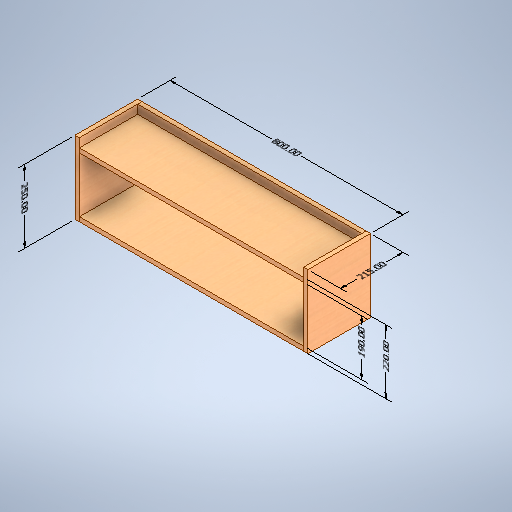
# Autodesk Inventor part: MM_00001.1.0
Saved by Autodesk Inventor 2025.3 (Build 293356000, 356)
## iProperties
Created: 2025-08-13
Part Number: MM_00001.1.0
Material: Wood (Cherry)
Document SubType Name: Modeling
Designer: FerreRo
Density: 0.63 g/cm^3
Appearance: Cherry - Natural Low Gloss
Author: FerreRo
Autodesk Inventor part; units mm, degrees
ref_plane "YZ Plane" through (0, 0, 0) normal (1, 0, 0) x (0, 1, 0)
ref_plane "XZ Plane" through (0, 0, 0) normal (0, 1, 0) x (-1, 0, 0)
ref_plane "XY Plane" through (0, 0, 0) normal (0, 0, 1) x (1, 0, 0)
sketch "Sketch1" plane through (0, 0, 0) normal (0, 0, 1) x (1, 0, 0)
  line L0 (-400, 125) -> (400, 125)
  line L1 (400, 125) -> (400, -125)
  line L2 (400, -125) -> (-400, -125)
  line L3 (-400, -125) -> (-400, 125)
  line L4 (-400, 125) -> (400, -125) construction
  line L5 (400, 125) -> (-400, -125) construction
  point P0 (0, 0)
  dimension "d0" = 800
  dimension "d1" = 250
  constraints: 12 end point, 2 midpoint, 2 parallel, 1 horizontal, 1 perpendicular
  measures "d0" distance of L1.end L2.end
  measures "d1" distance of L0.end L1.end
sketch "Sketch2" plane through (0, 0, 0) normal (0, 1, 0) x (-1, 0, 0)
  line L0 (400, -100) -> (-400, -100)
  line L1 (-400, -100) -> (-400, 100)
  line L2 (-400, 100) -> (400, 100)
  line L3 (400, 100) -> (400, -100)
  line L4 (400, -100) -> (-400, 100) construction
  line L5 (-400, -100) -> (400, 100) construction
  point P0 (0, 0)
  dimension "d2" = 800
  dimension "d3" = 200
  constraints: 12 end point, 2 midpoint, 2 parallel, 1 horizontal, 1 perpendicular
  measures "d2" distance of L1.end L2.end
  measures "d3" distance of L0.end L1.end
sketch "Sketch3" plane through (0, 0, 0) normal (0, 0, 1) x (1, 0, 0)
  line L0 (-400, -125) -> (-400, 125) construction
  line L1 (-400, 125) -> (-385, 125)
  line L2 (-385, 125) -> (-385, -125)
  line L3 (-385, -125) -> (-400, -125)
  line L4 (-400, -125) -> (-400, 125)
  point P0 (0, 0)
  dimension "d4" = 15
  constraints: 8 end point, 2 parallel, 1 collinear, 1 horizontal, 1 perpendicular
  measures "d4" distance of L1.start L1.end
extrude "Extrusion1" add sketch "Sketch3" along normal mid plane 200
move faces "Move1" translate (0, 0, -15) faces at (-395, 41.6667, -100)
mirror "Mirror1" about plane through (0, 0, 0) normal (1, 0, 0)
sketch "Sketch4" plane through (0, 0, 0) normal (0, 0, 1) x (1, 0, 0)
  line L0 (400, -125) -> (-400, -125) construction
  line L1 (-385, -125) -> (-385, 125) construction
  line L2 (385, -125) -> (385, 125) construction
  line L3 (-385, -125) -> (385, -125)
  line L4 (385, -125) -> (385, -110)
  line L5 (385, -110) -> (-385, -110)
  line L6 (-385, -110) -> (-385, -125)
  point P0 (0, 0)
  dimension "d7" = 15
  constraints: 8 end point, 2 parallel, 1 horizontal, 1 perpendicular, 1 point on line
  measures "d7" distance between parallel lines of L0 L5
extrude "Extrusion2" add sketch "Sketch4" along normal mid plane 200 separate body
pattern_linear "Rectangular Pattern1" count 2 spacing 205 along (0, 1, 0) bodies 2
sketch "Sketch5" plane through (0, 0, -100) normal (0, 0, -1) x (-1, 0, 0)
  line L0 (-385, 125) -> (-385, -125) construction
  line L1 (385, 125) -> (385, -125) construction
  line L2 (-385, -125) -> (385, -125) construction
  line L3 (-385, 125) -> (385, 125)
  line L4 (385, 125) -> (385, 35)
  line L5 (385, 35) -> (-385, 35)
  line L6 (-385, 35) -> (-385, 125)
  line L7 (-385, -125) -> (385, -125)
  line L8 (385, -125) -> (385, -35)
  line L9 (385, -35) -> (-385, -35)
  line L10 (-385, -35) -> (-385, -125)
  point P0 (0, 0)
  dimension "d16" = 90
  dimension "d17" = 90
  constraints: 16 end point, 4 parallel, 2 horizontal, 2 perpendicular, 2 point on line
  measures "d16" distance between parallel lines of L5 L3
  measures "d17" distance between parallel lines of L2 L9
extrude "Extrusion3" add sketch "Sketch5" along normal blind 15 separate body contours L10 L9 L8 L7
extrude "Extrusion4" add sketch "Sketch5" along normal blind 15 separate body contours L3 L4 L5 L6
equation "\"d5\" = d3"
equation "\"d8\" = d3"
equation "\"d17\" = d16"
equation "\"d18\" = d4"
equation "\"d20\" = d4"
